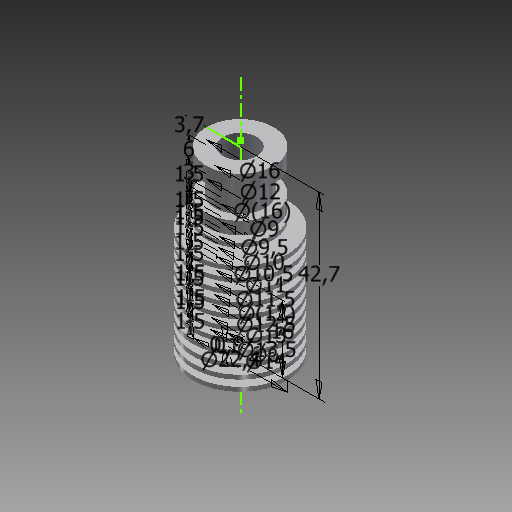
# Autodesk Inventor part: HeatSink
Saved by Autodesk Inventor 2017 SP1 (Build 210196100, 196)
## iProperties
Created: 2015-02-05
Part Number: HeatSink
Material: Типовые
Document SubType Name: Modeling
Designer: Parabolik
Density: 1 g/cm^3
Appearance: По умолчанию
Author: Parabolik
Autodesk Inventor part; units mm, degrees
ref_plane "YZ Plane" through (0, 0, 0) normal (1, 0, 0) x (0, 1, 0)
ref_plane "XZ Plane" through (0, 0, 0) normal (0, 1, 0) x (-1, 0, 0)
ref_plane "XY Plane" through (0, 0, 0) normal (0, 0, 1) x (1, 0, 0)
sketch "Эскиз1" plane through (0, 0, 0) normal (0, 0, 1) x (1, 0, 0)
  line L0 (0, 42.7) -> (-8, 42.7)
  line L1 (-8, 42.7) -> (-8, 39)
  line L2 (-8, 39) -> (-6, 39)
  line L3 (-6, 39) -> (-6, 33)
  line L4 (-6, 33) -> (-8, 33)
  line L5 (-8, 33) -> (-8, 30)
  line L6 (-8, 30) -> (-4.5, 30)
  line L7 (-4.5, 30) -> (-4.5, 28.5)
  line L8 (-4.5, 28.5) -> (-8, 28.5)
  line L9 (-8, 28.5) -> (-8, 27.5)
  line L10 (-8, 27.5) -> (-4.5, 27.5)
  line L11 (-4.5, 27.5) -> (-4.5, 26)
  line L12 (-4.5, 26) -> (-11.2, 26)
  line L13 (-11.2, 26) -> (-11.2, 25)
  line L14 (-11.2, 25) -> (-4.75, 25)
  line L15 (-4.75, 25) -> (-4.75, 23.5)
  line L16 (-4.75, 23.5) -> (-11.2, 23.5)
  line L17 (-11.2, 23.5) -> (-11.2, 22.5)
  line L18 (-11.2, 22.5) -> (-5, 22.5)
  line L19 (-5, 22.5) -> (-5, 21)
  line L20 (-5, 21) -> (-11.2, 21)
  line L21 (-11.2, 21) -> (-11.2, 20)
  line L22 (-11.2, 20) -> (-5.25, 20)
  line L23 (-5.25, 20) -> (-5.25, 18.5)
  line L24 (-11.2, 18.5) -> (-11.2, 17.5)
  line L25 (-11.2, 17.5) -> (-5.5, 17.5)
  line L26 (-5.5, 17.5) -> (-5.5, 16)
  line L27 (-5.5, 16) -> (-11.2, 16)
  line L28 (-11.2, 16) -> (-11.2, 15)
  line L29 (-11.2, 15) -> (-5.75, 15)
  line L30 (-5.75, 15) -> (-5.75, 13.5)
  line L31 (-5.75, 13.5) -> (-11.2, 13.5)
  line L32 (-11.2, 13.5) -> (-11.2, 12.5)
  line L33 (-11.2, 11) -> (-6, 11)
  line L34 (-11.2, 11) -> (-11.2, 10)
  line L35 (-11.2, 10) -> (-6.25, 10)
  line L36 (-6.25, 10) -> (-6.25, 8.5)
  line L37 (-6.25, 8.5) -> (-11.2, 8.5)
  line L38 (-11.2, 8.5) -> (-11.2, 7.5)
  line L39 (-6.5, 6) -> (-11.2, 6)
  line L40 (-11.2, 6) -> (-11.2, 5)
  line L41 (-11.2, 5) -> (-6.75, 5)
  line L42 (-6.75, 5) -> (-6.75, 3.5)
  line L43 (-6.75, 3.5) -> (-11.2, 3.5)
  line L44 (-11.2, 3.5) -> (-11.2, 2.5)
  line L45 (-11.2, 2.5) -> (-7, 2.5)
  line L46 (-7, 2.5) -> (-7, 1)
  line L47 (-7, 1) -> (-11.2, 1)
  line L48 (-11.2, 1) -> (-11.2, 0)
  line L49 (-11.2, 0) -> (-3, 0)
  line L50 (-5.25, 18.5) -> (-11.2, 18.5)
  line L51 (0, 57) -> (0, -13)
  line L52 (-11.2, 12.5) -> (-6, 12.5)
  line L53 (-6, 12.5) -> (-6, 11)
  line L54 (-11.2, 7.5) -> (-6.5, 7.5)
  line L55 (-6.5, 7.5) -> (-6.5, 6)
  line L56 (0, 42.7) -> (0, 16)
  line L57 (-3, 0) -> (-3, 16)
  line L58 (-3, 16) -> (0, 16)
  line L59 (-3, 0) -> (-3, -0.9)
  line L60 (-3.5, -0.4) -> (-3, 0)
  line L61 (-3.5, -0.4) -> (-3.5, -0.5)
  line L62 (-3.5, -0.5) -> (-3, -0.9)
  point P0 (0, 43.9)
  point P1 (0, 0)
  dimension "d13" = 1.5
  dimension "d14" = 1.5
  dimension "d15" = 1.5
  dimension "d16" = 1.5
  dimension "d17" = 1.5
  dimension "d18" = 1.5
  dimension "d19" = 3.7
  dimension "d20" = 6
  dimension "d21" = 3
  dimension "d32" = 16
  dimension "d33" = 12
  dimension "d34" = 1
  dimension "d35" = 1
  dimension "d36" = 1
  dimension "d37" = 1
  dimension "d38" = 1
  dimension "d39" = 1
  dimension "d40" = 1.5
  dimension "d43" = 1
  dimension "d44" = 1.5
  dimension "d47" = 1
  dimension "d48" = 1.5
  dimension "d49" = 1
  dimension "d50" = 1.5
  dimension "d51" = 1
  dimension "d52" = 22.4
  dimension "d53" = 16
  dimension "d54" = 9
  dimension "d55" = 9.5
  dimension "d56" = 10
  dimension "d57" = 10.5
  dimension "d58" = 11
  dimension "d61" = 12.5
  dimension "d63" = 13.5
  dimension "d64" = 14
  dimension "d66" = 11.5
  dimension "d67" = 1
  dimension "d68" = 12
  dimension "d69" = 13
  dimension "d70" = 1.5
  dimension "d71" = 1.5
  dimension "d99" = 42.7
  dimension "d118" = 16
  dimension "d119" = 6
  dimension "d131" = 0.9
  dimension "d133" = 0.1
  constraints: 127 end point, 28 point on line, 4 perpendicular, 3 vertical, 2 collinear, 2 horizontal
  measures "d13" distance between parallel lines of L27 L25
  measures "d14" distance between parallel lines of L50 L22
  measures "d15" distance between parallel lines of L20 L18
  measures "d16" distance between parallel lines of L16 L14
  measures "d17" distance between parallel lines of L12 L10
  measures "d18" distance between parallel lines of L8 L6
  measures "d19" distance between parallel lines of L2 L0
  measures "d20" distance between parallel lines of L4 L2
  measures "d21" distance between parallel lines of L6 L4
  measures "d32" diameter of L1 L51
  measures "d33" diameter of L3 L51
  measures "d34" distance between parallel lines of L10 L8
  measures "d35" distance between parallel lines of L14 L12
  measures "d36" distance between parallel lines of L18 L16
  measures "d37" distance between parallel lines of L22 L20
  measures "d38" distance between parallel lines of L25 L50
  measures "d39" distance between parallel lines of L29 L27
  measures "d40" distance between parallel lines of L31 L29
  measures "d43" distance between parallel lines of L35 L33
  measures "d44" distance between parallel lines of L37 L35
  measures "d47" distance between parallel lines of L41 L39
  measures "d48" distance between parallel lines of L43 L41
  measures "d49" distance between parallel lines of L45 L43
  measures "d50" distance between parallel lines of L47 L45
  measures "d51" distance between parallel lines of L49 L47
  measures "d52" diameter of L48 L51
  measures "d53" diameter of L5 L51
  measures "d54" diameter of L7 L51
  measures "d55" diameter of L15 L51
  measures "d56" diameter of L19 L51
  measures "d57" diameter of L23 L51
  measures "d58" diameter of L26 L51
  measures "d61" diameter of L36 L51
  measures "d63" diameter of L42 L51
  measures "d64" diameter of L46 L51
  measures "d66" diameter of L30 L51
  measures "d67" distance between parallel lines of L31 L52
  measures "d68" diameter of L53 L51
  measures "d69" diameter of L55 L51
  measures "d70" distance between parallel lines of L39 L54
  measures "d71" distance between parallel lines of L33 L52
  measures "d99" distance between parallel lines of L0 L49
  measures "d118" distance of L49.end L57.end
  measures "d119" diameter of L57 L51
  measures "d131" distance of L49.end L59.end
  measures "d133" distance of L60.start L61.end
revolve "Вращение1" add sketch "Эскиз1" angle 360 about axis through (0, 57, 0) along (0, -1, 0) contours L51 L58 L57 L49 L48 L47 L46 L45 L44 L43 L42 L41 L40 L39 L55 L54 L38 L37 L36 L35 L34 L33 L53 L52 L32 L31 L30 L29 L28 L27 L26 L25 L24 L50 L23 L22 L21 L20 L19 L18 L17 L16 L15 L14 L13 L12 L11 L10 L9 L8 L7 L6 L5 L4 L3 L2 L1 L0
sketch "Эскиз2" plane through (0, 0, 0) normal (0, -1, 0) x (1, 0, 0)
  point P0 (0, 0)
  point P1 (0, 0)
  point P2 (0, 0)
  constraints: 1 coincident
hole "Отверстие1" at (0, 0, 0) direction (0, 1, 0) diameter 4 end through all
hole "Отверстие3" at (0, 0, 0) direction (0, 1, 0) diameter 5.917 depth 16 tip angle 118 thread size "M7x1" class "6H" standard "ISO Metric profile"
sketch "Эскиз3" plane through (0, 42.7, 0) normal (0, 1, 0) x (1, 0, 0)
  point P0 (0, 0)
  point P1 (0, 0)
  constraints: 1 coincident
hole "Отверстие4" at (0, 42.7, 0) direction (0, -1, 0) diameter 8 depth 8 tip angle 118
coil "Пружина3" sketch "Эскиз1" operation cut axis through (0, 57, 0) along (0, 1, 0) pitch 1 turns 11 hand right contours L59 L62 L61 L60
